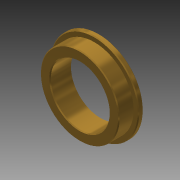
# Autodesk Inventor part: Ball Shifting Bushing
Saved by Autodesk Inventor 2013 (Build 170138000, 138)
## iProperties
Created: 2013-06-04
Part Number: Ball Shifting Bushing
Material: Brass, Soft Yellow
Document SubType Name: Modeling
Designer: mvarma
Density: 1 g/cm^3
Author: mvarma
Autodesk Inventor part; units mm, degrees
ref_plane "YZ Plane" through (0, 0, 0) normal (1, 0, 0) x (0, 1, 0)
ref_plane "XZ Plane" through (0, 0, 0) normal (0, 1, 0) x (-1, 0, 0)
ref_plane "XY Plane" through (0, 0, 0) normal (0, 0, 1) x (1, 0, 0)
sketch "Sketch1" plane through (0, 0, 0) normal (0, 0, 1) x (1, 0, 0)
  circle A0 centre (0, 0) radius 9.525
  circle A1 centre (0, 0) radius 12.7
  circle A2 centre (0, 0) radius 14.2875
  dimension "d0" = 19.05
  dimension "d1" = 25.4
  dimension "d2" = 28.575
  constraints: 3 centre point, 3 coincident
  measures "d0" diameter of A0
  measures "d1" diameter of A1
  measures "d2" diameter of A2
extrude "Extrusion1" add sketch "Sketch1" along normal blind 4.7625 contours A1
extrude "Extrusion2" add sketch "Sketch1" against normal blind 1.5875 contours A1 | A2
chamfer "Chamfer1" distance 0.254 angle 45 4 edges at (-12.7, 0, 4.7625) (-9.525, 0, 4.7625) (-14.2875, 0, 0) (-14.2875, 0, -1.5875)
sketch "Sketch2" plane through (0, 0, -1.5875) normal (0, 0, -1) x (-1, 0, 0)
  circle A0 centre (0, 0) radius 9.525 projected
  circle A1 centre (0, 0) radius 14.2875 projected
  circle A2 centre (0, 0) radius 10.3188
  dimension "d10" = 20.6375
  constraints: 1 centre point, 1 coincident
  measures "d10" diameter of A2
extrude "Extrusion3" add sketch "Sketch2" along normal blind 0.3969 contours A2
body "Solid1"
